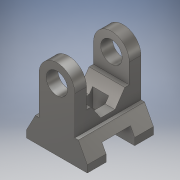
# Autodesk Inventor part: FORK127
Saved by Autodesk Inventor 2018 (Build 220112000, 112)
## iProperties
Created: 2017-10-05
Part Number: FORK127
Material: Stainless Steel
Document SubType Name: Modeling
Designer: kurtis
Density: 8 g/cm^3
Appearance: Semi-Polished
Author: kurtis
Autodesk Inventor part; units mm, degrees
ref_plane "YZ Plane" through (0, 0, 0) normal (1, 0, 0) x (0, 1, 0)
ref_plane "XZ Plane" through (0, 0, 0) normal (0, 1, 0) x (-1, 0, 0)
ref_plane "XY Plane" through (0, 0, 0) normal (0, 0, 1) x (1, 0, 0)
sketch "Sketch1" plane through (0, 0, 0) normal (0, 0, 1) x (1, 0, 0)
  line L0 (0, 0) -> (0, 70) construction
  circle A0 centre (0, 70) radius 12
  arc A1 (20, 70) -> (-20, 70) centre (0, 70) ccw
  line L1 (0, 0) -> (34, 0)
  line L2 (0, 0) -> (-34, 0)
  line L3 (-34, 0) -> (-34, 8)
  line L4 (34, 0) -> (34, 8)
  line L5 (0, 0) -> (0, 0) construction
  line L6 (20, 27) -> (24, 27)
  line L7 (-20, 27) -> (-24, 27)
  line L8 (-24, 27) -> (-34, 8)
  line L9 (24, 27) -> (34, 8)
  line L10 (20, 70) -> (20, 27)
  line L11 (-20, 70) -> (-20, 27)
  line L12 (0, 0) -> (0, 17) construction
  line L13 (0, 17) -> (-9, 17)
  line L14 (0, 17) -> (9, 17)
  line L15 (0, 17) -> (9, 17) construction
  line L16 (9, 17) -> (9, 42.3642)
  line L17 (9, 42.3642) -> (-9, 42.3642)
  line L18 (-9, 42.3642) -> (-9, 17)
  dimension "d0" = 70
  dimension "d1" = 24
  dimension "d2" = 20
  dimension "d3" = 34
  dimension "d4" = 34
  dimension "d5" = 8
  dimension "d6" = 8
  dimension "d10" = 4
  dimension "d11" = 4
  dimension "d14" = 19
  dimension "d15" = 19
  dimension "d34" = 17
  dimension "d35" = 9
  dimension "d39" = 18
  constraints: 38 end point, 8 perpendicular, 4 horizontal, 2 centre point, 2 coincident, 2 point on circle, 2 point on line, 2 tangent, 2 vertical, 1 collinear, 1 parallel
  measures "d0" distance of L0.start L0.end
  measures "d1" diameter of A0
  measures "d2" radius of A1
  measures "d3" distance of L0.start L1.end
  measures "d4" distance of L0.start L2.end
  measures "d5" distance of L2.end L3.end
  measures "d6" distance of L1.end L4.end
  measures "d10" distance of L7.start L7.end
  measures "d11" distance of L6.start L6.end
  measures "d14" vertical distance of L4.end L6.end
  measures "d15" vertical distance of L3.end L7.end
  measures "d34" distance of L0.start L12.end
  measures "d35" distance of L12.end L13.end
  measures "d39" distance of L16.end L17.end
extrude "Extrusion1" add sketch "Sketch1" along normal mid plane 74 contours L10 L6 L9 L4 L1 L2 L3 L8 L7 L11 A1 | L13 L18 L17 L16 L14
sketch "Sketch2" plane through (34, 0, 37) normal (1, 0, 0) x (0, 0, -1)
  line L0 (37, 0) -> (53, 0)
  line L1 (74, 0) -> (0, 0) projected
  line L2 (37, 0) -> (21, 0)
  line L3 (21, 0) -> (21, 17)
  line L4 (21, 17) -> (53, 17)
  line L5 (53, 17) -> (53, 0)
  line L6 (0, 0) -> (29, 0) construction
  line L7 (29, 32) -> (45, 32)
  line L8 (0, 0) -> (18, 0) construction
  line L9 (18, 48) -> (56, 48) construction
  line L10 (56, 48) -> (45, 32)
  line L11 (29, 32) -> (18, 48)
  line L12 (74, 90) -> (0, 90) projected
  line L13 (0, 90) -> (13, 90)
  line L14 (13, 90) -> (13, 48)
  line L15 (74, 90) -> (61, 90)
  line L16 (61, 90) -> (61, 48)
  line L17 (18, 48) -> (13, 48)
  line L18 (56, 48) -> (61, 48)
  line L19 (13, 90) -> (61, 90)
  line L20 (0, 27) -> (0, 70) projected
  line L21 (74, 70) -> (74, 27) projected
  dimension "d23" = 32
  dimension "d24" = 16
  dimension "d27" = 38
  dimension "d45" = 32
  dimension "d46" = 17
  dimension "d47" = 13
  dimension "d48" = 13
  dimension "d49" = 5
  dimension "d50" = 16
  dimension "d58" = 11
  dimension "d69" = 48
  dimension "d70" = 21
  dimension "d72" = 56
  dimension "d73" = 74
  constraints: 36 end point, 5 perpendicular, 5 point on line, 3 horizontal, 2 collinear, 1 midpoint, 1 parallel
  measures "d23" distance of L6.end L7.start
  measures "d24" distance of L7.start L7.end
  measures "d27" distance of L9.start L9.end
  measures "d45" distance between parallel lines of L5 L3
  measures "d46" distance between parallel lines of L0 L4
  measures "d47" distance between parallel lines of L20 L14
  measures "d48" distance between parallel lines of L21 L16
  measures "d49" distance of L9.end L16.end
  measures "d50" distance between parallel lines of L18 L7
  measures "d58" horizontal distance of L9.end L7.end
  measures "d69" distance between parallel lines of L1 L18
  measures "d70" distance between parallel lines of L5 L21
  measures "d72" distance from line of L8.end L21
  measures "d73" distance from line of L13.start L21
extrude "Extrusion2" cut sketch "Sketch2" against normal blind 84
extrude "Extrusion3" cut sketch "Sketch1" along normal mid plane 24 contours L13 L18 L17 L16 L14
equation "\"d5\" = d6"
equation "\"d15\" = d14"
body "Solid1"
